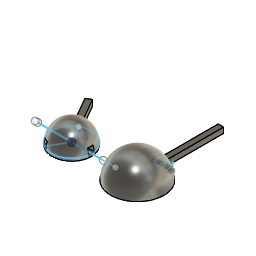
animometer v2 Krum (Autodesk Fusion 360 design; units mm, degrees)
Autodesk Fusion 360 part; units mm, degrees
note: some values were not read from the file. Chosen so that the rebuilt part matches the saved one: which face or edge a step refers to; which pieces of a blend or face edit are solid.
sphere "SpherePrimitive1" add diameter 39 placed x (1, 0, 0) y (0, 1, 0) z (0, 0, 1) at (0, 0, 0) makes body 1
sketch "Sketch2" plane through (0, 0, 0) normal (0, 1, 0) x (1, 0, 0)
  line L0 (32.2582, 0) -> (-26.919, 0)
  constraint horizontal L0
split "Split1" by curves path "Sketch2" along L0 bodies 1 makes body 2 at (-9.6666, -16.743, -2.5453)
delete_body "RemoveBody1" bodies 2
shell "Shell1" thickness 1 removed faces 1 at (-7.6576, 4.4211, 0) on bodies 1
box "BoxPrimitive1" add length 4 width 4 height 43 placed x (0, 0, 1) y (1, 0, 0) z (0, 1, 0) at (0, 0, 0) separate body makes body 3
move_body "Move1" bodies 3 to x (1, 0, 0) y (0, 1, 0) z (0, 0, 1) at (-2, 0, 0)
move_body "Move2" bodies 3 to x (1, 0, 0) y (0, 1, 0) z (0, 0, 1) at (0, 18.4866, 0)
combine "Combine1" operation add target body 3 tool bodies 1
move_body "Move3" bodies 3 to x (1, 0, 0) y (0, 1, 0) z (0, 0, 1) at (48.3199, 0, 0)
sphere "SpherePrimitive2" add diameter 29 placed x (1, 0, 0) y (0, 1, 0) z (0, 0, 1) at (0, 0, 0) separate body makes body 4
sketch "Sketch5" plane through (0, 0, 0) normal (0, 1, 0) x (1, 0, 0)
sketch "Sketch6" plane through (0, 0, 0) normal (0, 1, 0) x (1, 0, 0)
  line L0 (23.2236, 0) -> (-25.1454, 0)
  constraint horizontal L0
split "Split2" by curves path "Sketch6" along L0 bodies 4 makes body 5 at (-7.188, -12.4499, -1.8926)
delete_body "RemoveBody2" bodies 5
shell "Shell2" thickness 14.2604 removed faces 1 at (-1.5019, -8.021, 0) on bodies 4
cylinder "CylinderPrimitive1" add diameter 12.4 height 1 placed x (1, 0, 0) y (0, 1, 0) z (0, 0, 1) at (0, 0, 0) separate body makes body 6
move_face "OffsetFaces1" offset 12.0423 1 faces at (1.6068, 0.7965, 1) on bodies 6
move_face "OffsetFaces2" offset 3 1 faces at (1.6068, 0.7965, 0) on bodies 6
combine "Combine2" operation add target body 6 tool bodies 4
cylinder "CylinderPrimitive2" cut diameter 9.8 height -5.5 placed x (0, 1, 0) y (1, 0, 0) z (0, 0, -1) at (0, 0, -3) bodies 6
cylinder "CylinderPrimitive3" cut diameter 4.2 height 6.505 placed x (1, 0, 0) y (0, 1, 0) z (0, 0, 1) at (-8.9888, 0, 0) bodies 6
move_face "MoveFace1" to x (1, 0, 0) y (0, 1, 0) z (0, 0, 1) at (-0.0942, 0, 0) 1 faces at (-6.8992, -0.2091, 2.1683) on bodies 6
move_face "MoveFace2" to x (1, 0, 0) y (0, 1, 0) z (0, 0, 1) at (-0.17, 0, 0) 1 faces at (-6.9934, -0.2091, 2.1683) on bodies 6
move_face "OffsetFaces3" offset -0.1 1 faces at (-7.1634, -0.2091, 2.1683) on bodies 6
move_face "OffsetFaces4" offset 0.65 1 faces at (-8.6715, -0.3062, 6.505) on bodies 6
cylinder "CylinderPrimitive4" cut diameter 8.3 height 11.002 placed x (1, 0, 0) y (0, 1, 0) z (0, 0, 1) at (0, 0, 0) bodies 6
sketch "Sketch11" plane through (0, 0, 0) normal (0, 0, 1) x (1, 0, 0)
  circle A0 centre (0, 0) radius 14.4916
  line L0 (0, 0) -> (14.4916, 0)
  line L1 (0, 0) -> (-7.2453, -12.5503)
  line L2 (0, 0) -> (-7.2453, 12.5503)
  constraint coincident A0.centre L0.start
  constraint coincident A0 L0.end
  constraint horizontal L0
  constraint coincident A0 L2.end
  constraint coincident A0 L1.end
box "BoxPrimitive2" add length 4.1 width 4.1 height 27.9003 placed x (0, 0, -1) y (-1, 0, 0) z (0, 1, 0) at (4.1, 0, 0) separate body makes body 7
move_body "Move4" bodies 7 to x (0.866025, 0.5, 0) y (-0.5, 0.866025, 0) z (0, 0, 1) at (-5.0211, 4.5968, 4.0887)
copy_body "CopyPasteBodies1" bodies 7 makes body 8
box "BoxPrimitive3" add length 4.1 width 4.1 height -26.9343 placed x (0, 0, 1) y (1, 0, 0) z (0, 1, 0) at (-4.1, 0, 0) separate body makes body 9
move_body "Move5" bodies 9 to x (0.866025, -0.5, 0) y (0.5, 0.866025, 0) z (0, 0, 1) at (-1.4699, -6.6471, 0)
box "BoxPrimitive4" add length 4.1 width 4.1 height 28.597 placed x (0, 0, 1) y (0, -1, 0) z (1, 0, 0) at (0, 0, 0) separate body makes body 10
move_body "Move6" bodies 10 to x (1, 0, 0) y (0, 1, 0) z (0, 0, 1) at (6.4913, 2.0498, 0)
sketch "Sketch16" plane through (0, 0, 0) normal (0, 0, 1) x (1, 0, 0)
move_face "OffsetFaces5" offset 1 1 faces at (6.4913, -0.6836, 1.3667) on bodies 10
move_face "OffsetFaces6" offset 1 1 faces at (-2.6535, -5.9638, 1.3667) on bodies 9
move_face "OffsetFaces7" offset 2 1 faces at (-8.6222, -4.6019, 0) on bodies 6
combine "Combine3" operation cut target body 6 tool bodies 10
combine "Combine4" operation cut target body 6 tool bodies 7
combine "Combine5" operation cut target body 6 tool bodies 9
move_face "OffsetFaces8" offset 0.863 1 faces at (-2.1535, -5.0978, 1.3667) on bodies 6
move_face "OffsetFaces9" offset -0.137 1 faces at (-3.8375, 5.2801, 2.7221) on bodies 6
move_face "OffsetFaces10" offset 0.863 1 faces at (5.4913, -0.6836, 1.3667) on bodies 6
ref_plane "WorkPlane1" through (50.023, 0, 0) normal (1, 0, 0) x (0, 1, 0)
sketch "Sketch17" plane through (0, 0, 0) normal (0, 0, 1) x (1, 0, 0)
  spline S0 degree 5 poles (46.32, 19.395) (46.2543, 19.3912) (46.1207, 19.3822) (45.9134, 19.3642) (45.6232, 19.3312) (45.2359, 19.2739) (44.8222, 19.1994) (44.3803, 19.1066) (43.9102, 18.9954) (43.4139, 18.8671) (42.8936, 18.7231) (42.46, 18.5967) (42.1256, 18.4958) (41.8987, 18.426) (41.7842, 18.3904) knots 0 0 0 0 0 0 0.1 0.2 0.3 0.4 0.5 0.6 0.7 0.8 0.9 1 1 1 1 1 1
  line L0 (41.7842, 18.3904) -> (46.3035, 24.2859)
  line L1 (46.3035, 24.2859) -> (46.32, 19.395)
  spline S1 degree 5 poles (50.3, 19.4) (50.3904, 19.3914) (50.571, 19.3734) (50.8415, 19.3434) (51.2013, 19.2976) (51.6495, 19.23) (52.0961, 19.1512) (52.5408, 19.0601) (52.9836, 18.9564) (53.4246, 18.8404) (53.8639, 18.7133) (54.2141, 18.6033) (54.4762, 18.5164) (54.6506, 18.4566) (54.7377, 18.4262) knots 0 0 0 0 0 0 0.1 0.2 0.3 0.4 0.5 0.6 0.7 0.8 0.9 1 1 1 1 1 1
  line L2 (54.7377, 18.4262) -> (50.297, 24.4012)
  line L3 (50.297, 24.4012) -> (50.3, 19.4)
  point P0 (44.5521, 19.1411)
  point P1 (52.5354, 19.058)
extrude "Extrude1" add sketch "Sketch17" along normal blind 1.5 separate body contours S1 L2 L3 makes body 11
move_body "Move7" bodies 11 to x (1, 0, 0) y (0, 1, 0) z (0, 0, 1) at (0, 0, 1.1944)
extrude "Extrude2" add sketch "Sketch17" along normal blind 1.5 separate body contours S0 L0 L1 makes body 12
move_body "Move8" bodies 12 to x (1, 0, 0) y (0, 1, 0) z (0, 0, 1) at (0, 0, 1.1109)
move_body "Move9" bodies 12 to x (1, 0, 0) y (0, 1, 0) z (0, 0, 1) at (0, -0.2019, 0)
combine "Combine6" operation add target body 3 tool bodies 12
extrude "Extrude3" cut 1 faces at (5.739, -0.4301, -3) along direction (0, 0, 1) blind 1.0292 on bodies 6 bodies 6
delete_body "RemoveBody3" bodies 11
